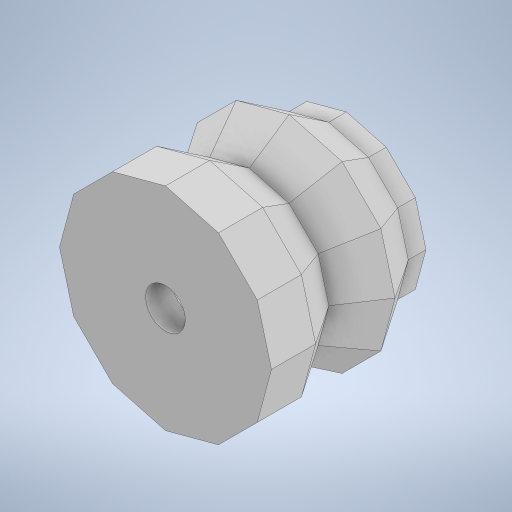
# Autodesk Inventor part: Test9
Saved by Autodesk Inventor 2023 (Build 270158000, 158)
## iProperties
Created: 2024-07-03
Part Number: Test9
Material: 일반
Document SubType Name: Modeling
Designer: ojs08
Density: 1 g/cm^3
Appearance: 기본값
Author: ojs08
Autodesk Inventor part; units mm, degrees
ref_plane "YZ Plane" through (0, 0, 0) normal (1, 0, 0) x (0, 1, 0)
ref_plane "XZ Plane" through (0, 0, 0) normal (0, 1, 0) x (-1, 0, 0)
sketch "스케치1" plane through (0, 0, 0) normal (0, 0, 1) x (1, 0, 0)
  line L0 (10.392305, 6) -> (12, 0)
  line L1 (12, 0) -> (10.392305, -6)
  line L2 (10.392305, -6) -> (6, -10.392305)
  line L3 (6, -10.392305) -> (0, -12)
  line L4 (0, -12) -> (-6, -10.392305)
  line L5 (-6, -10.392305) -> (-10.392305, -6)
  line L6 (-10.392305, -6) -> (-12, 0)
  line L7 (-12, 0) -> (-10.392305, 6)
  line L8 (-10.392305, 6) -> (-6, 10.392305)
  line L9 (-6, 10.392305) -> (0, 12)
  line L10 (0, 12) -> (6, 10.392305)
  line L11 (6, 10.392305) -> (10.392305, 6)
  line L12 (-16.8, 0) -> (16.8, 0)
  point P0 (0, 0)
  point P1 (0, 0)
  dimension "d0" = 24
  constraints: 24 end point, 1 coincident, 1 point on line, 25 other
  measures "d0" distance of L0.end L6.end
ref_plane "작업 평면1" through (0, 0, 4.5) normal (0, 0, 1) x (1, 0, 0)
sketch "스케치2" plane through (0, 0, 4.5) normal (0, 0, 1) x (1, 0, 0)
  line L0 (0, -12.6) -> (0, 12.6)
  line L1 (4.5, -7.794229) -> (0, -9)
  line L2 (0, -9) -> (-4.5, -7.794229)
  line L3 (-4.5, -7.794229) -> (-7.794229, -4.5)
  line L4 (-7.794229, -4.5) -> (-9, 0)
  line L5 (-9, 0) -> (-7.794229, 4.5)
  line L6 (-7.794229, 4.5) -> (-4.5, 7.794229)
  line L7 (-4.5, 7.794229) -> (0, 9)
  line L8 (0, 9) -> (4.5, 7.794229)
  line L9 (4.5, 7.794229) -> (7.794229, 4.5)
  line L10 (7.794229, 4.5) -> (9, 0)
  line L11 (9, 0) -> (7.794229, -4.5)
  line L12 (7.794229, -4.5) -> (4.5, -7.794229)
  point P0 (0, 0)
  point P1 (0, 0)
  dimension "d2" = 18
  constraints: 24 end point, 1 coincident, 1 point on line, 25 other
  measures "d2" distance of L1.end L7.end
loft "로프트1" add profiles "스케치1", "스케치2"
mirror "미러1" about plane through (0, 0, 4.5) normal (0, 0, 1) of "로프트1"
mirror "미러2" about plane through (0, 0, 0) normal (0, 0, -1) of "로프트1"
sketch "스케치3" plane through (12, 0, 9) normal (0, 0, 1) x (0.9659258, 0.258819, 0)
  line L0 (0, 6.211657) -> (0, 0)
  line L1 (-3.105829, 11.59111) -> (0, 6.211657)
  line L2 (-8.485281, 14.696938) -> (-3.105829, 11.59111)
  line L3 (-14.696938, 14.696938) -> (-8.485281, 14.696938)
  line L4 (-20.076391, 11.59111) -> (-14.696938, 14.696938)
  line L5 (-23.18222, 6.211657) -> (-20.076391, 11.59111)
  line L6 (-23.18222, 0) -> (-23.18222, 6.211657)
  line L7 (-20.076391, -5.379453) -> (-23.18222, 0)
  line L8 (-14.696938, -8.485281) -> (-20.076391, -5.379453)
  line L9 (-8.485281, -8.485281) -> (-14.696938, -8.485281)
  line L10 (-3.105829, -5.379453) -> (-8.485281, -8.485281)
  line L11 (0, 0) -> (-3.105829, -5.379453)
  point P0 (-11.59111, 3.105829)
extrude "돌출1" add sketch "스케치3" along normal blind 2.5
shell "쉘1" thickness 0.5 removed faces 0 ; own thickness 2 on faces at (8.184186, -6.842093, -1.5) (3.666667, -10.01752, -1.5) (-1.833333, -10.50876, -1.5) (-6.842093, -8.184186, -1.5) (-10.01752, -3.666667, -1.5) (-10.50876, 1.833333, -1.5) (-8.184186, 6.842093, -1.5) (10.50876, -1.833333, -1.5) (10.01752, 3.666667, -1.5) (6.842093, 8.184186, -1.5) (1.833333, 10.50876, -1.5) (-3.666667, 10.01752, -1.5) (-6.842093, -8.184186, 7.5) (-10.01752, -3.666667, 7.5) (-10.50876, 1.833333, 7.5) (-8.184186, 6.842093, 7.5) (-3.666667, 10.01752, 7.5) (1.833333, 10.50876, 7.5) (6.842093, 8.184186, 7.5) (10.01752, 3.666667, 7.5) (-1.833333, -10.50876, 7.5) (3.666667, -10.01752, 7.5) (8.184186, -6.842093, 7.5) (10.50876, -1.833333, 7.5)
sketch "스케치4" plane through (12, 0, 11.5) normal (0, 0, 1) x (0.9659258, 0.258819, 0)
  line L0 (-3.105829, 11.59111) -> (-8.485281, 14.696938)
  line L1 (-8.485281, 14.696938) -> (-14.696938, 14.696938)
  line L2 (-14.696938, 14.696938) -> (-20.076391, 11.59111)
  line L3 (-20.076391, 11.59111) -> (-23.18222, 6.211657)
  line L4 (-23.18222, 6.211657) -> (-23.18222, 0)
  line L5 (-23.18222, 0) -> (-20.076391, -5.379453)
  line L6 (-20.076391, -5.379453) -> (-14.696938, -8.485281)
  line L7 (-14.696938, -8.485281) -> (-8.485281, -8.485281)
  line L8 (-8.485281, -8.485281) -> (-3.105829, -5.379453)
  line L9 (-3.105829, -5.379453) -> (0, 0)
  line L10 (0, 0) -> (0, 6.211657)
  line L11 (0, 6.211657) -> (-3.105829, 11.59111)
  point P0 (-11.59111, 3.105829)
extrude "돌출2" add sketch "스케치4" along normal blind 2.5
sketch "스케치5" plane through (12, 0, 14) normal (0, 0, 1) x (0.9659258, 0.258819, 0)
  circle A0 centre (-11.59111, 3.105829) radius 2.25
  point P0 (-11.59111, 3.105829)
  dimension "d13" = 4.5
  constraints: 1 centre point, 1 coincident
  measures "d13" diameter of A0
extrude "돌출3" cut sketch "스케치5" against normal blind 3
sketch "스케치6" plane through (9, 0, -4.5) normal (0, 0, -1) x (-0.9659258, -0.258819, 0)
  circle A0 centre (8.693332, 2.329371) radius 2.25
  line L0 (0, 4.658743) -> (0, 0)
  line L1 (0, 0) -> (2.329371, -4.03459)
  line L2 (2.329371, -4.03459) -> (6.363961, -6.363961)
  line L3 (6.363961, -6.363961) -> (11.022704, -6.363961)
  line L4 (11.022704, -6.363961) -> (15.057293, -4.03459)
  line L5 (15.057293, -4.03459) -> (17.386665, 0)
  line L6 (17.386665, 0) -> (17.386665, 4.658743)
  line L7 (17.386665, 4.658743) -> (15.057293, 8.693332)
  line L8 (15.057293, 8.693332) -> (11.022704, 11.022704)
  line L9 (11.022704, 11.022704) -> (6.363961, 11.022704)
  line L10 (6.363961, 11.022704) -> (2.329371, 8.693332)
  line L11 (2.329371, 8.693332) -> (0, 4.658743)
  point P0 (8.693332, 2.329371)
extrude "돌출4" add sketch "스케치6" along normal blind 2 contours A0 | L11 L10 L9 L8 L7 L6 L5 L4 L3 L2 L1 L0
